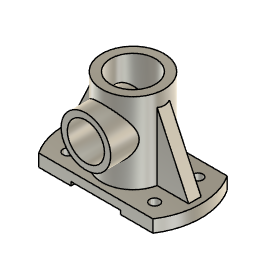
15 (Autodesk Fusion 360 design; units mm, degrees)
Autodesk Fusion 360 part; units mm, degrees
sketch "草图1" plane through (0, 0, 0) normal (0, 0, 1) x (1, 0, 0)
  line L0 (-46.0977, 30) -> (46.0977, 30)
  line L1 (-46.0977, -30) -> (46.0977, -30)
  line L2 (-130, 0) -> (170, 0) construction
  line L3 (0, 120) -> (0, -120) construction
  circle A0 centre (-35, 17.5) radius 4
  circle A1 centre (35, 17.5) radius 4
  circle A2 centre (35, -17.5) radius 4
  circle A3 centre (-35, -17.5) radius 4
  arc A4 (46.0977, -30) -> (46.0977, 30) centre (0, 0) ccw
  arc A5 (-46.0977, 30) -> (-46.0977, -30) centre (0, 0) ccw
  dimension "d1" = 110
  dimension "d2" = 60
  dimension "d3" = 8
  dimension "d4" = 35
  dimension "d5" = 70
  constraint coincident A4.centre A5.centre
  constraint coincident L0.start A4
  constraint horizontal L0
  constraint horizontal L1
  constraint horizontal L2
  constraint vertical L3
  constraint equal L0 L1
  constraint symmetric L3 A0 A1
  constraint symmetric L3 A2 A3
  constraint symmetric L2 A0 A3
  constraint concentric A4 A5
  measures "d1" diameter of A4
  measures "d2" vertical distance of L0.start L1.start
  measures "d3" diameter of A1
  measures "d4" distance of A1.centre A2.centre
  measures "d5" distance of A2.centre A3.centre
extrude "拉伸1" add sketch "草图1" against normal blind 10 makes body 1
sketch "草图2" plane through (0, -30, 0) normal (0, -1, 0) x (1, 0, 0)
  line L0 (46.0977, 0) -> (-46.0977, 0)
  line L1 (-46.0977, 0) -> (-46.0977, -10)
  line L2 (-46.0977, -10) -> (46.0977, -10)
  line L3 (46.0977, -10) -> (46.0977, 0)
  line L4 (-46.0977, 0) -> (46.0977, 0)
  line L5 (46.0977, 0) -> (46.0977, -10)
  line L6 (46.0977, -10) -> (-46.0977, -10)
  line L7 (-46.0977, -10) -> (-46.0977, 0)
  line L8 (-20, -7) -> (20, -7)
  line L9 (20, -7) -> (20, -10)
  line L10 (20, -10) -> (-20, -10)
  line L11 (-20, -10) -> (-20, -7)
  line L12 (0, 5) -> (0, -26.915) construction
  dimension "d8" = 40
  dimension "d9" = 3
  constraint horizontal L4
  constraint vertical L5
  constraint horizontal L6
  constraint vertical L7
  constraint coincident L2.end L3.start
  constraint coincident L0.end L1.start
  constraint horizontal L8
  constraint vertical L9
  constraint horizontal L10
  constraint vertical L11
  constraint coincident L2 L9.end
  constraint perpendicular L4 L12
  constraint symmetric L9 L11 L12
  measures "d8" distance of L9.end L10.end
  measures "d9" distance of L8.end L9.end
extrude "拉伸2" cut sketch "草图2" against normal blind 80 contours L2 L6 L8 L9 L10 L11 bodies 1
sketch "草图3" plane through (0, 0, 0) normal (0, 0, 1) x (-1, 0, 0)
  circle A0 centre (35, 17.5) radius 4
  circle A1 centre (-35, -17.5) radius 4
  circle A2 centre (35, -17.5) radius 4
  circle A3 centre (-35, 17.5) radius 4
  arc A4 (46.0977, -30) -> (46.0977, 30) centre (0, 0) ccw
  line L0 (46.0977, 30) -> (-46.0977, 30)
  arc A5 (-46.0977, 30) -> (-46.0977, -30) centre (0, 0) ccw
  line L1 (-46.0977, -30) -> (46.0977, -30)
  circle A6 centre (0, 0) radius 25
  circle A7 centre (0, 0) radius 18
  dimension "d12" = 50
  dimension "d13" = 36
  constraint coincident A4.centre A5.centre
  constraint concentric A6 A7
  measures "d12" diameter of A6
  measures "d13" diameter of A7
extrude "拉伸3" cut sketch "草图3" against normal blind 45 contours A7 bodies 1
extrude "拉伸4" add sketch "草图3" along normal blind 65 contours A6 bodies 1
sketch "草图4" plane through (0, 0, 0) normal (0, 1, 0) x (1, 0, 0)
  circle A0 centre (0, -35) radius 20
  circle A1 centre (0, -35) radius 15
  line L0 (-25, -65) -> (25, -65)
  dimension "d18" = 40
  dimension "d19" = 30
  dimension "d20" = 30
  constraint concentric A0 A1
  measures "d18" diameter of A0
  measures "d19" diameter of A1
  measures "d20" distance of A0.centre L0
extrude "拉伸5" add sketch "草图4" against normal blind 38 bodies 1
extrude "拉伸6" cut sketch "草图4" against normal blind 60 contours A1 bodies 1
sketch "草图5" plane through (0, 0, 0) normal (0, 1, 0) x (1, 0, 0)
  line L0 (50, 0) -> (19.69, -65)
  line L1 (-19.69, -65) -> (-50, 0)
  line L2 (-19.69, -65) -> (-19.69, 0)
  line L3 (19.69, -65) -> (19.69, 0)
  line L4 (-60, 0) -> (-19.69, 0) construction
  line L5 (19.69, 0) -> (60, 0) construction
  line L6 (-50, 0) -> (-19.69, 0)
  line L7 (19.69, 0) -> (50, 0)
  dimension "d25" = 100
  dimension "d26" = 65
  constraint horizontal L6
  constraint collinear L4 L6
  constraint coincident L3.end L6
  constraint perpendicular L2 L6
  constraint perpendicular L3 L6
  constraint collinear L4 L5
  constraint collinear L6 L7
  measures "d25" distance of L1.end L0.start
  measures "d26" angle of L0 L6
extrude "拉伸7" add sketch "草图5" along normal mid plane 10 separate body makes body 2 at (-29.7933, 5, 21.6667) makes body 3 at (29.7933, 5, 21.6667)
combine "合并1" operation add target body 1 tool bodies 3 2
